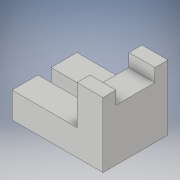
# Autodesk Inventor part: Part2
Saved by Autodesk Inventor 2018 (Build 220112000, 112)
## iProperties
Created: 2020-01-07
Part Number: Part2
Material: Generic
Document SubType Name: Modeling
Designer: AOFUser
Density: 1 g/cm^3
Appearance: Default
Author: AOFUser
Autodesk Inventor part; units mm, degrees
ref_plane "YZ Plane" through (0, 0, 0) normal (1, 0, 0) x (0, 1, 0)
ref_plane "XZ Plane" through (0, 0, 0) normal (0, 1, 0) x (-1, 0, 0)
ref_plane "XY Plane" through (0, 0, 0) normal (0, 0, 1) x (1, 0, 0)
sketch "Sketch1" plane through (0, 0, 0) normal (0, 1, 0) x (-1, 0, 0)
  line L0 (0, 0) -> (-88.9, 0)
  line L1 (-88.9, 0) -> (-88.9, -63.5)
  line L2 (-88.9, -63.5) -> (0, -63.5)
  line L3 (0, -63.5) -> (0, 0)
  dimension "d0" = 88.9
  dimension "d1" = 63.5
  constraints: 8 end point, 2 parallel, 1 horizontal, 1 perpendicular
  measures "d0" distance of L2.end L1.end
  measures "d1" distance of L1.end L0.end
extrude "Extrusion1" add sketch "Sketch1" along normal blind 25.4
sketch "Sketch2" plane through (0, 25.4, 0) normal (0, 1, 0) x (1, 0, 0)
  line L0 (88.9, 63.5) -> (0, 63.5) projected
  line L1 (0, 63.5) -> (0, 38.1)
  line L2 (0, 63.5) -> (0, 0) projected
  line L3 (0, 38.1) -> (38.1, 38.1)
  line L4 (38.1, 38.1) -> (38.1, 25.4)
  line L5 (38.1, 25.4) -> (0, 25.4)
  line L6 (0, 25.4) -> (0, 38.1)
  dimension "d4" = 25.4
  dimension "d5" = 38.1
  dimension "d6" = 12.7
  constraints: 10 end point, 2 parallel, 1 horizontal, 1 perpendicular, 1 point on line
  measures "d4" distance of L0.end L1.end
  measures "d5" distance of L4.end L5.end
  measures "d6" distance of L3.end L4.end
extrude "Extrusion2" cut sketch "Sketch2" against normal blind 25.4
sketch "Sketch3" plane through (0, 25.4, 0) normal (0, 1, 0) x (1, 0, 0)
  line L0 (88.9, 63.5) -> (0, 63.5) projected
  line L1 (0, 0) -> (88.9, 0) projected
  line L2 (88.9, 63.5) -> (63.5, 63.5)
  line L3 (63.5, 63.5) -> (63.5, 0)
  line L4 (63.5, 0) -> (88.9, 0)
  line L5 (88.9, 0) -> (88.9, 63.5)
  dimension "d9" = 25.4
  constraints: 8 end point, 2 parallel, 1 horizontal, 1 perpendicular, 1 point on line
  measures "d9" distance of L4.end L3.end
extrude "Extrusion3" add sketch "Sketch3" along normal blind 38.1
sketch "Sketch4" plane through (0, 63.5, 0) normal (0, 1, 0) x (1, 0, 0)
  line L0 (88.9, 63.5) -> (0, 63.5) projected
  line L1 (88.9, 63.5) -> (88.9, 50.8)
  line L2 (88.9, 0) -> (88.9, 63.5) projected
  line L3 (63.5, 63.5) -> (63.5, 0) projected
  line L4 (88.9, 50.8) -> (63.5, 50.8)
  line L5 (63.5, 50.8) -> (63.5, 12.7)
  line L6 (63.5, 12.7) -> (88.9, 12.7)
  line L7 (88.9, 12.7) -> (88.9, 50.8)
  point P0 (0, 0)
  dimension "d12" = 12.7
  dimension "d13" = 38.1
  constraints: 10 end point, 2 parallel, 2 point on line, 1 horizontal, 1 perpendicular
  measures "d12" distance of L0.start L1.end
  measures "d13" distance of L5.end L4.end
extrude "Extrusion4" cut sketch "Sketch4" against normal blind 12.7 contours L2 L6 L3 L4
body "Solid1"
